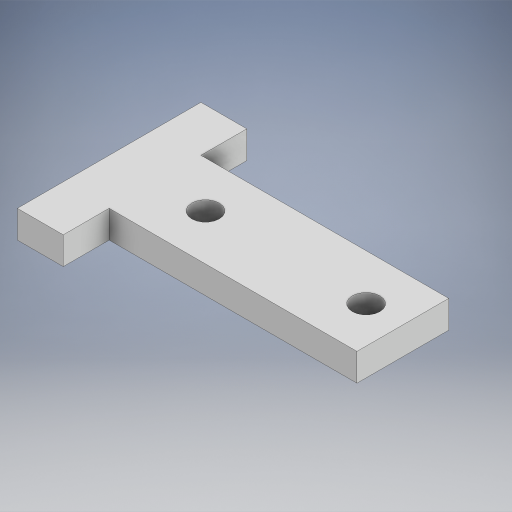
# Autodesk Inventor part: Stand T Sd Serayu 2024
Saved by Autodesk Inventor 2024 (Build 280153000, 153)
## iProperties
Created: 2024-07-09
Part Number: Stand T Sd Serayu 2024
Material: Generic
Document SubType Name: Modeling
Designer: LENOVO
Density: 1 g/cm^3
Appearance: Default
Author: LENOVO
Autodesk Inventor part; units mm, degrees
ref_plane "YZ Plane" through (0, 0, 0) normal (1, 0, 0) x (0, 1, 0)
ref_plane "XZ Plane" through (0, 0, 0) normal (0, 1, 0) x (-1, 0, 0)
ref_plane "XY Plane" through (0, 0, 0) normal (0, 0, 1) x (1, 0, 0)
sketch "Sketch1" plane through (0, 0, 0) normal (0, 1, 0) x (-1, 0, 0)
  line L0 (16, 10) -> (-16, 10)
  line L1 (-16, 10) -> (-16, -10)
  line L2 (-16, -10) -> (16, -10)
  line L3 (16, -10) -> (16, 10)
  line L4 (16, 10) -> (-16, -10) construction
  line L5 (-16, 10) -> (16, -10) construction
  line L6 (-16, -10) -> (11, -10)
  line L7 (11, -10) -> (11, -5)
  line L8 (11, -5) -> (-16, -5)
  line L9 (-16, -5) -> (-16, -10)
  line L10 (-16, 10) -> (11, 10)
  line L11 (11, 10) -> (11, 5)
  line L12 (11, 5) -> (-16, 5)
  line L13 (-16, 5) -> (-16, 10)
  line L14 (11, 0) -> (8, 0)
  line L15 (8, 0) -> (5.5, 0)
  line L16 (5.5, 0) -> (-12, 0)
  circle A0 centre (5.5, 0) radius 1.5
  circle A1 centre (-12, 0) radius 1.5
  point P0 (0, 0)
  dimension "d0" = 32
  dimension "d1" = 20
  dimension "d2" = 27
  dimension "d3" = 5
  dimension "d4" = 27
  dimension "d5" = 5
  dimension "d6" = 3
  dimension "d7" = 2.5
  dimension "d8" = 17.5
  dimension "d9" = 3
  dimension "d10" = 3
  constraints: 34 end point, 6 parallel, 4 horizontal, 3 perpendicular, 2 centre point, 2 coincident, 2 midpoint, 2 point on line
  measures "d0" distance of L2.end L1.end
  measures "d1" distance of L1.end L0.end
  measures "d2" distance of L8.end L7.end
  measures "d3" distance of L7.end L6.end
  measures "d4" distance of L11.end L12.end
  measures "d5" distance of L10.end L11.end
  measures "d6" distance of L14.start L14.end
  measures "d7" distance of L14.end L15.end
  measures "d8" distance of L15.end L16.end
  measures "d9" diameter of A0
  measures "d10" diameter of A1
extrude "Extrusion1" add sketch "Sketch1" along normal blind 3 contours L3 L2 L7 L8 L1 L12 L11 L0
body "Solid1"
